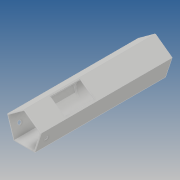
# Autodesk Inventor part: hull
Saved by Autodesk Inventor 2019 (Build 230136000, 136)
## iProperties
Created: 2019-03-09
Part Number: hull
Material: Générique
Document SubType Name: Modeling
Designer: Theo
Density: 1 g/cm^3
Appearance: Par défaut
Author: Theo
Autodesk Inventor part; units mm, degrees
ref_plane "YZ Plane" through (0, 0, 0) normal (1, 0, 0) x (0, 1, 0)
ref_plane "XZ Plane" through (0, 0, 0) normal (0, 1, 0) x (-1, 0, 0)
sketch "Esquisse2" plane through (0, 0, 0) normal (0, 0, 1) x (1, 0, 0)
  line L0 (11.62468, -16) -> (-11.62468, -16)
  line L1 (-11.62468, -16) -> (-18.809128, 6.111456)
  line L2 (-18.809128, 6.111456) -> (0, 19.777088)
  line L3 (0, 19.777088) -> (18.809128, 6.111456)
  line L4 (18.809128, 6.111456) -> (11.62468, -16)
  line L5 (19.984699, 6.493422) -> (12.351223, -17)
  line L6 (12.351223, -17) -> (-12.351223, -17)
  line L7 (-12.351223, -17) -> (-19.984699, 6.493422)
  line L8 (-19.984699, 6.493422) -> (0, 21.013156)
  line L9 (0, 21.013156) -> (19.984699, 6.493422)
  point P0 (0, 0)
  point P1 (0, 0)
  point P2 (0, 0)
  dimension "d9" = 16
  dimension "d10" = 1
  constraints: 20 end point, 2 coincident, 1 horizontal, 1 parallel, 22 other
  measures "d9" distance from line of L0 point (0, 0)
  measures "d10" distance between parallel lines of L0 L6
extrude "Extrusion2" add sketch "Esquisse2" along normal blind 150
sketch "Esquisse3" plane through (-12.351223, -17, 0) normal (-0.9510565, -0.309017, 0) x (0, 0, 1)
  line L0 (0, 12.351223) -> (150, 12.351223)
  line L1 (0, 0) -> (0, 24.702446)
  line L2 (0, 0) -> (150, 0)
  line L3 (150, 24.702446) -> (150, 0)
  line L4 (0, 24.702446) -> (150, 24.702446)
  point P0 (140, 12.351223)
  dimension "d23" = 10
  constraints: 1 horizontal alignment, 1 midpoint, 1 point on line
  measures "d23" distance from line of L3 point (140, 12.351)
hole "Perçage1" at (-16.167961, -5.253289, 140) direction (0.9510565, 0.309017, 0) diameter 4.5 depth 1 clearance for "Vis à tête plate fraisée ISO 2009/7046" size "M4" standard "ISO"
mirror "Symétrie1" about plane through (0, 0, 0) normal (1, 0, 0) of "Perçage1"
ref_plane "Plan de construction1" through (0, 0, 75) normal (0, 0, 1) x (1, 0, 0)
sketch "Esquisse4" plane through (0, 0, 75) normal (0, 0, 1) x (1, 0, 0)
  line L0 (-11.62468, -16) -> (-18.809128, 6.111456)
  line L1 (-18.809128, 6.111456) -> (0, 19.777088)
  line L2 (0, 19.777088) -> (18.809128, 6.111456)
  line L3 (18.809128, 6.111456) -> (11.62468, -16)
  line L4 (11.62468, -16) -> (-11.62468, -16)
  line L5 (12.351223, -17) -> (19.984699, 6.493422)
  line L6 (19.984699, 6.493422) -> (0, 21.013156)
  line L7 (0, 21.013156) -> (-19.984699, 6.493422)
  line L8 (-19.984699, 6.493422) -> (-12.351223, -17)
  line L9 (-12.351223, -17) -> (12.351223, -17)
  circle A0 centre (0, 0) radius 15
  dimension "d25" = 30
  constraints: 1 centre point, 1 coincident
  measures "d25" diameter of A0
extrude "Extrusion3" add sketch "Esquisse4" against normal up to surface (75 mm away) contours L0 L1 L2 L3 L4
sketch "Esquisse5" plane through (0, 0, 0) normal (0, 0, -1) x (-1, 0, 0)
  circle A0 centre (0, 0) radius 15
  line L0 (-19.984699, 6.493422) -> (-12.351223, -17)
  line L1 (-12.351223, -17) -> (12.351223, -17)
  line L2 (12.351223, -17) -> (19.984699, 6.493422)
  line L3 (19.984699, 6.493422) -> (0, 21.013156)
  line L4 (0, 21.013156) -> (-19.984699, 6.493422)
extrude "Extrusion4" add sketch "Esquisse5" along normal blind 5 contours A0 | L4 L3 L2 L1 L0
chamfer "Chanfrein1" distance 1 angle 45 1 edges at (-15, 0, 0)
sketch "Esquisse6" plane through (-19.984699, 6.493422, 150) normal (-0.5877853, 0.809017, 0) x (0.809017, 0.5877853, 0)
  line L0 (27.351223, 75) -> (-2.648777, 75)
  line L1 (-6.457905, 75) -> (0.726543, 75)
  line L2 (12.351223, 75) -> (-6.457905, 75)
  line L3 (31.160351, 75) -> (12.351223, 75)
  line L4 (23.975903, 75) -> (31.160351, 75)
  line L5 (0.726543, 75) -> (23.975903, 75)
  line L6 (15.601223, 74) -> (9.101223, 74)
  line L7 (9.101223, 74) -> (9.101223, 37)
  line L8 (9.101223, 37) -> (15.601223, 37)
  line L9 (15.601223, 37) -> (15.601223, 74)
  line L10 (24.702446, 0) -> (0, 0)
  point P0 (12.351223, 150)
  point P1 (12.351223, 74)
  point P2 (12.351223, 75)
  dimension "d33" = 6.5
  dimension "d34" = 1
  dimension "d35" = 37
  constraints: 8 end point, 2 midpoint, 2 parallel, 1 horizontal, 1 perpendicular, 1 vertical alignment
  measures "d33" distance of L6.start L6.end
  measures "d34" distance between parallel lines of L0 L6
  measures "d35" distance between parallel lines of L8 L10
extrude "Extrusion5" [suppressed]
sketch "Esquisse8" plane through (-7.363044, 15.663591, 106) normal (-0.809017, -0.5877853, 0) x (0, 0, 1)
  line L0 (37, -1) -> (0, -1) projected
  line L1 (37, 0) -> (37, -1) projected
  line L2 (0, 0) -> (37, 0) projected
  line L3 (0, 0) -> (0, -1) projected
  line L4 (37, 7.5) -> (30.5, 7.5)
  line L5 (30.5, 7.5) -> (30.5, -8.5)
  line L6 (30.5, -8.5) -> (37, -8.5)
  line L7 (37, -8.5) -> (37, 7.5)
  point P0 (-106, -17)
  point P1 (37, -0.5)
  dimension "d40" = 6.5
  dimension "d41" = 16
  constraints: 8 end point, 2 midpoint, 2 parallel, 1 horizontal, 1 perpendicular
  measures "d40" distance of L4.start L4.end
  measures "d41" distance of L4.end L5.end
feature "Hélicoïde1" [suppressed]
fillet "Congé1" [suppressed]
fillet "Congé2" [suppressed]
sketch "Esquisse12" plane through (0, 21.013156, 150) normal (0.5877853, 0.809017, 0) x (0.809017, -0.5877853, 0)
  line L0 (0, 0) -> (0, 155)
  line L1 (24.702446, 0) -> (0, 0)
  line L2 (24.702446, 155) -> (24.702446, 0)
  line L3 (0, 155) -> (24.702446, 155)
  line L4 (2, 30) -> (22, 30)
  line L5 (22, 30) -> (22, 65)
  line L6 (22, 65) -> (2, 65)
  line L7 (2, 65) -> (2, 30)
  point P0 (12.351223, 150)
  dimension "d71" = 30
  dimension "d72" = 35
  dimension "d73" = 2
  dimension "d75" = 20
  constraints: 8 end point, 2 parallel, 1 horizontal, 1 perpendicular
  measures "d71" distance between parallel lines of L4 L1
  measures "d72" distance between parallel lines of L6 L4
  measures "d73" distance between parallel lines of L0 L7
  measures "d75" distance between parallel lines of L7 L5
extrude "Extrusion8" cut sketch "Esquisse12" against normal up to surface (1 mm away) contours L7 L6 L5 L4
sketch "Esquisse14" plane through (0, 0, 75) normal (0, 0, 1) x (1, 0, 0)
  circle A0 centre (0, 0) radius 15
  line L0 (-11.62468, -16) -> (-18.809128, 6.111456)
  line L1 (11.62468, -16) -> (-11.62468, -16)
  line L2 (18.809128, 6.111456) -> (11.62468, -16)
  line L3 (0, 19.777088) -> (18.809128, 6.111456)
  line L4 (-18.809128, 6.111456) -> (0, 19.777088)
  line L5 (-16.276555, -4.919072) -> (-15.517053, -7.256578)
  line L6 (-15.517053, -7.256578) -> (-14.666402, -6.638544)
  line L7 (-14.666402, -6.638544) -> (-15.413013, -4.340711)
  line L8 (-7.363044, 15.663591) -> (-9.790095, 13.900235)
  line L9 (-9.790095, 13.900235) -> (-9.20231, 13.091218)
  line L10 (-9.20231, 13.091218) -> (-6.775259, 14.854574)
  line L11 (-6.775259, 14.854574) -> (-7.363044, 15.663591)
  line L12 (17.210589, 7.272863) -> (1.030249, 19.028568)
  line L13 (17.798374, 8.08188) -> (17.210589, 7.272863)
  line L14 (1.618034, 19.837585) -> (17.798374, 8.08188)
  line L15 (1.618034, 19.837585) -> (1.030249, 19.028568)
  line L16 (17.210589, 7.272863) -> (14.573734, -3.550533)
  line L17 (-5.275259, 15.944388) -> (1.030249, 19.028568)
  line L18 (-14.666402, -6.638544) -> (-10.486502, -10.725357)
  arc A1 (-10.486502, -10.725357) -> (14.573734, -3.550533) centre (0, 0) ccw
  line L19 (-14.666402, -6.638544) -> (-11.62468, -16)
  line L20 (11.62468, -16) -> (-11.62468, -16)
  line L21 (11.62468, -16) -> (18.809128, 6.111456)
  line L22 (17.210589, 7.272863) -> (18.809128, 6.111456)
  line L23 (-5.275259, 15.944388) -> (0, 19.777088)
  line L24 (1.030249, 19.028568) -> (0, 19.777088)
  dimension "d82" = 1.5
  constraints: 18 end point, 4 collinear, 4 point on circle, 2 tangent, 1 centre point, 1 coincident, 1 horizontal, 1 point on line, 1 other
  measures "d82" horizontal distance of L10.end L17.start
extrude "Extrusion10" add sketch "Esquisse14" along normal blind 45 contours A0 L16 L3 L2 L1 L0 L18 | L17 L4 L3
chamfer "Chanfrein3" distance 1 angle 45 2 edges at (-5.8182, 13.8257, 75) (14.8931, -1.788, 75)
chamfer "Chanfrein4" distance 1 angle 45 5 edges at (9.9923, 13.7533, -5) (-9.9923, 13.7533, -5) (-16.168, -5.2533, -5) (0, -17, -5) (16.168, -5.2533, -5)
chamfer "Chanfrein5" distance 0.5 angle 45 9 edges at (1.618, 19.8376, 102.5) (9.7082, 13.9597, 85) (9.7082, 13.9597, 120) (17.7984, 8.0819, 102.5) (9.9923, 13.7533, 150) (-9.9923, 13.7533, 150) (-16.168, -5.2533, 150) (0, -17, 150) (16.168, -5.2533, 150)
sketch "Esquisse17" plane through (0, 0, -5) normal (0, 0, -1) x (-1, 0, 0)
  point P0 (0, 0)
  point P1 (0, 0)
  constraints: 1 coincident
hole "Perçage2" at (0, 0, -5) direction (0, 0, 1) diameter 18.917 depth 5 thread size "M20x1" class "6H" standard "ISO Metric profile"
